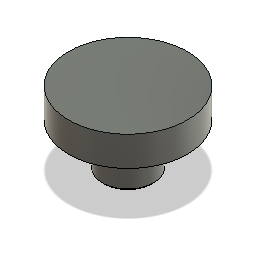
part for Braun Bowl (Autodesk Fusion 360 design; units mm, degrees)
Autodesk Fusion 360 part; units mm, degrees
sketch "Sketch2" plane through (0, 0, 0) normal (0, 1, 0) x (1, 0, 0)
  circle A0 centre (0, 0) radius 15
  dimension "d1" = 30
  constraint coincident A0.centre origin
  measures "d1" diameter of A0
extrude "Extrude1" add sketch "Sketch2" along normal blind 9
sketch "Sketch3" plane through (0, 0, 0) normal (0, -1, 0) x (1, 0, 0)
  circle A0 centre (0, 0) radius 15
  circle A1 centre (0, 0) radius 7.5
  dimension "d4" = 15
  constraint coincident A0.centre A1.centre
  measures "d4" diameter of A1
extrude "Extrude2" add sketch "Sketch3" along normal blind 11 contours A1
chamfer "Chamfer1" distance 0.5 angle 45 1 edges at (-6.9925, -11, -2.7121)
sketch "Sketch4" plane through (0, -11, 0) normal (0, -1, 0) x (1, 0, 0)
  circle A0 centre (0, 0) radius 7
  circle A1 centre (0, 0) radius 3.5
  dimension "d8" = 7
  constraint coincident A0.centre A1.centre
  measures "d8" diameter of A1
extrude "Extrude3" cut sketch "Sketch4" against normal blind 14 contours A1
extrude "Extrude4" cut 1 faces at (3.8315, 9, -5.6199) along direction (0, -1, 0) blind 1.5
sketch "Sketch5" plane through (0, 7.5, 0) normal (0, 1, 0) x (-1, 0, 0)
  circle A0 centre (0, 0) radius 15
move_face "OffsetFaces1" offset -1 1 faces at (7.4907, -7, -0.3738)
chamfer "Chamfer2" distance 0.5 angle 45 1 edges at (-6.0601, 0, 2.3505)
